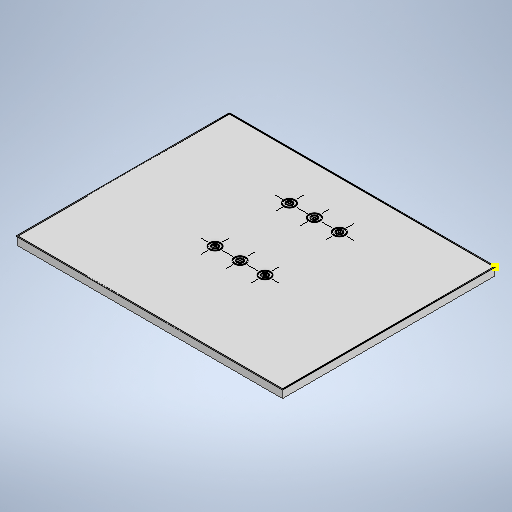
# Autodesk Inventor part: CAM_axis_6_bottom_frame(bottom)
Saved by Autodesk Inventor 2025.2 (Build 292293000, 293)
## iProperties
Created: 2025-08-09
Part Number: CAM_axis_6_bottom_frame(bottom)
Material: Generic
Document SubType Name: Modeling
Designer: User
Density: 1 g/cm^3
Appearance: Default
Author: User
Autodesk Inventor part; units mm, degrees
ref_plane "YZ Plane" through (0, 0, 0) normal (1, 0, 0) x (0, 1, 0)
ref_plane "XZ Plane" through (0, 0, 0) normal (0, 1, 0) x (-1, 0, 0)
ref_plane "XY Plane" through (0, 0, 0) normal (0, 0, 1) x (1, 0, 0)
sketch "Sketch1" plane through (0, 0, 0) normal (0, 1, 0) x (-1, 0, 0)
  circle A0 centre (59.405, 18) radius 2
  circle A1 centre (50, 18) radius 2
  circle A2 centre (40.595, 18) radius 2
  circle A3 centre (40.595, 46) radius 2
  circle A4 centre (50, 46) radius 2
  circle A5 centre (59.405, 46) radius 2
  circle A6 centre (59.405, 18) radius 1.05
  circle A7 centre (50, 18) radius 1.05
  circle A8 centre (40.595, 18) radius 1.05
  circle A9 centre (40.595, 46) radius 1.05
  circle A10 centre (50, 46) radius 1.05
  circle A11 centre (59.405, 46) radius 1.05
  line L0 (100, 80) -> (100, 0)
  line L1 (0, 80) -> (100, 80)
  line L2 (0, 0) -> (0, 80)
  line L3 (100, 0) -> (0, 0)
  constraints: 12 centre point, 10 equal radius, 8 end point, 2 horizontal, 2 perpendicular, 2 vertical, 1 parallel, 23 other
extrude "Extrusion1" add sketch "Sketch1" against normal blind 3 contours A0 | A1 | A2 | A3 | A4 | A5 | L0 L3 L2 L1
body "Solid1"
